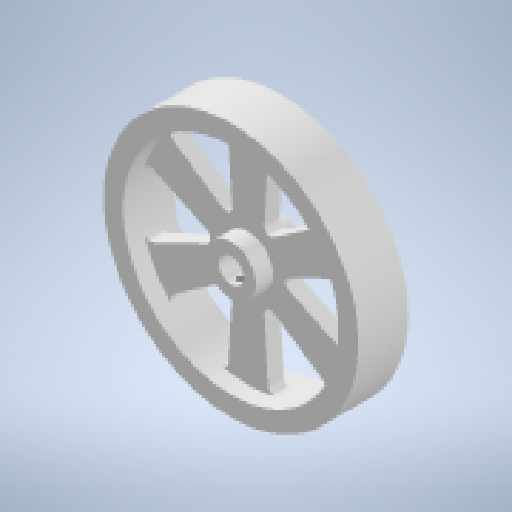
# Autodesk Inventor part: flywheel
Saved by Autodesk Inventor 2025.3 (Build 293356000, 356)
## iProperties
Created: 2019-03-25
Part Number: flywheel
Material: Generic
Document SubType Name: Modeling
Designer: ebolton
Manufacturer: Standard
Standards Organization: Custom
Density: 1 g/cm^3
Appearance: Default
PartAngTol0: 0.50 deg
PartAngTol1: 0.50 deg
PartAngTol2: 0.50 deg
PartLinTol0: 0.01 in
PartLinTol1: 0.01 in
PartLinTol2: 0.01 in
PartLinTol3: 0.005 in
PartAngTol3: 0deg30'
Author: ebolton
Autodesk Inventor part; units mm, degrees
ref_plane "YZ Plane (RIGHT)" through (0, 0, 0) normal (1, 0, 0) x (0, 1, 0)
ref_plane "XY Plane (FRONT)" through (0, 0, 0) normal (0, 0, 1) x (1, 0, 0)
sketch "Sketch2" plane through (0, 0, 0) normal (0, 0, 1) x (1, 0, 0)
  circle A0 centre (0, 0) radius 3.175
  circle A1 centre (0, 0) radius 6.35
  dimension "d0" = 6.35
  dimension "d1" = 12.7
  constraints: 2 centre point, 2 coincident
  measures "d0" diameter of A0
  measures "d1" diameter of A1
extrude "Extrusion1" add sketch "Sketch2" along normal mid plane 12.7
sketch "Sketch3" plane through (0, 0, 0) normal (0, 0, 1) x (1, 0, 0)
  circle A0 centre (0, 0) radius 27.5
  circle A1 centre (0, 0) radius 3.175 projected
  circle A2 centre (0, 0) radius 6.35
  circle A3 centre (0, 0) radius 6.35 projected
  dimension "d4" = 55
  constraints: 2 centre point, 2 coincident, 1 concentric
  measures "d4" diameter of A0
extrude "Extrusion2" add sketch "Sketch3" along normal mid plane 3.9688 contours A0
sketch "Sketch4" plane through (0, 0, 0) normal (0, 0, 1) x (1, 0, 0)
  circle A0 centre (0, 0) radius 3.175 projected
  circle A1 centre (0, 0) radius 32.5
  circle A2 centre (0, 0) radius 27.5
  circle A3 centre (0, 0) radius 27.5 projected
  dimension "d7" = 65
  constraints: 2 centre point, 2 coincident, 1 concentric
  measures "d7" diameter of A1
extrude "Extrusion3" add sketch "Sketch4" along normal mid plane 12.7 contours A1
sketch "Sketch7" plane through (0, 0, 1.9844) normal (0, 0, 1) x (1, 0, 0)
  circle A0 centre (0, 0) radius 3.175 construction
  line L0 (0, 0) -> (-6.7066, 25.0296) construction
  arc A1 (-5.1236, 25.1478) -> (-7.1175, 26.563) centre (-6.7066, 25.0296) ccw
  circle A2 centre (0, 0) radius 27.5 projected
  line L1 (0, 0) -> (0, 17.8508) construction
  arc A3 (-6.8709, 8.7338) -> (-3.9732, 9.7419) centre (-5.5563, 9.6237) ccw
  line L2 (0, 0) -> (-5.5563, 9.6237) construction
  circle A4 centre (0, 0) radius 11.1125 construction
  arc A5 (-19.4454, 19.4454) -> (-19.2168, 17.011) centre (-18.3229, 18.3229) ccw
  line L3 (-18.3229, 18.3229) -> (0, 0) construction
  line L4 (-19.2168, 17.011) -> (-6.4502, 8.3118)
  line L5 (-5.1236, 25.1478) -> (-3.9732, 9.7419)
  arc A6 (-7.1175, 26.563) -> (-19.4454, 19.4454) centre (0, 0) ccw
  dimension "d17" = 3.175
  dimension "d18" = 15
  dimension "d19" = 30
  dimension "d20" = 22.225
  dimension "d21" = 30
  constraints: 12 end point, 11 point on circle, 6 tangent, 5 centre point, 3 equal radius, 2 coincident, 1 concentric, 1 vertical
  measures "d17" diameter of A1
  measures "d18" angle of L1 L0
  measures "d19" angle of L1 L2
  measures "d20" diameter of A4
  measures "d21" angle of L0 L3
extrude "Extrusion4" cut sketch "Sketch7" along normal through all both and the other way through all contours L5 A3 L4 A5 A2 A1 picked at (-13.8134, 15.9498)
pattern_circular "Circular Pattern1" count 6 over 360 about axis through (0, 0, 0) along (0, 0, 1) of "Extrusion4"
ref_plane "Work Plane1" through (0, -6.35, 0) normal (0, 1, 0) x (-1, 0, 0)
sketch "Sketch8" plane through (0, -6.35, 0) normal (0, 1, 0) x (-1, 0, 0)
  line L0 (-16.7863, 6.35) -> (14.809, 6.35) construction
  point P0 (0, 0)
  dimension "d27" = 6.35
  constraints: 2 end point, 1 horizontal
  measures "d27" distance from line of L0 point (0, 0)
ref_plane "Work Plane2" through (16.7863, -6.35, 6.35) normal (0, -0.9397, 0.342) x (1, 0, 0)
sketch "Sketch9" plane through (16.7863, -6.35, 6.35) normal (0, -0.9397, 0.342) x (1, 0, 0)
  point P0 (-16.7863, -3.7952)
  point P1 (-16.7863, -1.2552)
  dimension "d29" = 2.54
  measures "d29" distance of point (-16.786, -3.795) point (-16.786, -1.255)
hole "Hole1" at (0, -6.7793, 5.1705) direction (0, 0.9397, -0.342) diameter 1.9304 depth 7.62 tip angle 118
body "Solid1"
